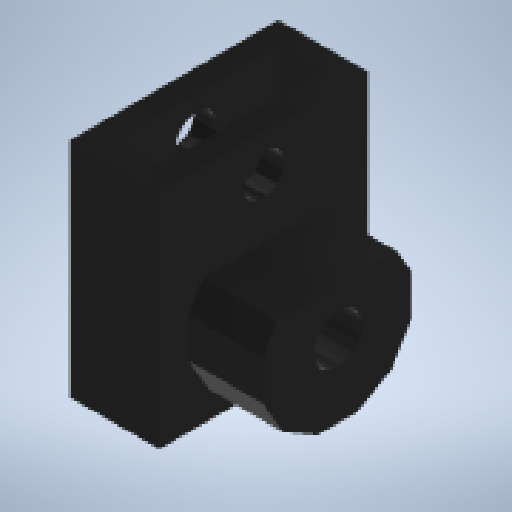
# Autodesk Inventor part: RollY
Saved by Autodesk Inventor 2023 (Build 270158000, 158)
## iProperties
Created: 2023-10-26
Part Number: RollY
Material: Thermoplastic Resin
Document SubType Name: Modeling
Designer: Mustapha
Density: 1.28 g/cm^3
Appearance: Smooth - Black
Mass: 11.287 g
Surface Area: 53.7238 cm^2
Volume: 8.81798 cm^3
Author: Mustapha
Autodesk Inventor part; units mm, degrees
ref_plane "YZ Plane" through (0, 0, 0) normal (1, 0, 0) x (0, 1, 0)
ref_plane "XZ Plane" through (0, 0, 0) normal (0, 1, 0) x (-1, 0, 0)
ref_plane "XY Plane" through (0, 0, 0) normal (0, 0, 1) x (1, 0, 0)
sketch "Sketch1" plane through (0, 0, 0) normal (0, 1, 0) x (-1, 0, 0)
  line L0 (0, 0) -> (6, 0)
  line L1 (6, 0) -> (6, -22)
  line L2 (6, -22) -> (0, -22)
  line L3 (0, -22) -> (0, 0)
  line L4 (9, 3) -> (-3, 3)
  line L5 (-3, 3) -> (-3, -25)
  line L6 (-3, -25) -> (9, -25)
  line L7 (9, -25) -> (9, 3)
  point P0 (3, 0)
  point P1 (3, -25)
  dimension "d0" = 22
  dimension "d1" = 6
  dimension "d2" = 3
  dimension "d3" = 3
  dimension "d4" = 3
  dimension "d5" = 3
  constraints: 16 end point, 4 parallel, 2 horizontal, 2 midpoint, 2 perpendicular
  measures "d0" distance between parallel lines of L2 L0
  measures "d1" distance between parallel lines of L3 L1
  measures "d2" distance from line of L4 point (3, 0)
  measures "d3" distance from line of point (3, -25) L2
  measures "d4" distance between parallel lines of L1 L7
  measures "d5" distance between parallel lines of L5 L3
extrude "Extrusion1" add sketch "Sketch1" along normal blind 30
sketch "Sketch2" plane through (3, 0, 3) normal (1, 0, 0) x (0, 0, -1)
  circle A0 centre (14, 25) radius 2.75
  line L0 (0, 30) -> (28, 30) projected
  point P0 (3, 0)
  dimension "d8" = 5.5
  dimension "d11" = 5
  constraints: 1 centre point
  measures "d8" diameter of A0
  measures "d11" distance from line of A0.centre L0
extrude "Extrusion2" cut sketch "Sketch2" against normal blind 30
sketch "Sketch3" plane through (3, 0, 3) normal (1, 0, 0) x (0, 0, -1)
  line L0 (6.6175, 3.6795) -> (3.938, 8.3205)
  line L1 (3.938, 8.3205) -> (3.938, 13.6795)
  line L2 (3.938, 13.6795) -> (6.6175, 18.3205)
  line L3 (6.6175, 18.3205) -> (11.2585, 21)
  line L4 (11.2585, 21) -> (16.6175, 21)
  line L5 (16.6175, 21) -> (21.2585, 18.3205)
  line L6 (21.2585, 18.3205) -> (23.938, 13.6795)
  line L7 (23.938, 13.6795) -> (23.938, 8.3205)
  line L8 (23.938, 8.3205) -> (21.2585, 3.6795)
  line L9 (21.2585, 3.6795) -> (16.6175, 1)
  line L10 (16.6175, 1) -> (11.2585, 1)
  line L11 (11.2585, 1) -> (6.6175, 3.6795)
  line L12 (0, 30) -> (28, 30) projected
  circle A0 centre (14, 10.8347) radius 3.253
  point P0 (3, 0)
  point P1 (13.938, 11)
  dimension "d12" = 10
  dimension "d13" = 19
  constraints: 24 end point, 1 centre point, 1 parallel, 25 other
  measures "d12" vertical distance of point (13.938, 11) L4.end
  measures "d13" distance from line of L12 point (13.938, 11)
extrude "Extrusion3" add sketch "Sketch3" along normal blind 10
sketch "Sketch5" plane through (3, 10.8347, -11) normal (1, 0, 0) x (0, 0, -1)
  circle A0 centre (0, 0) radius 1.5
  point P0 (-11, -10.8347)
  dimension "d18" = 3
  constraints: 1 centre point
  measures "d18" diameter of A0
extrude "Extrusion5" cut sketch "Sketch5" against normal blind 12
sketch "Sketch6" plane through (13, 0, 3) normal (1, 0, 0) x (0, 0, -1)
  line L0 (23, 22) -> (5, 22)
  line L1 (5, 22) -> (5, 17)
  line L2 (5, 17) -> (23, 17)
  line L3 (23, 17) -> (23, 22)
  line L4 (28, 0) -> (28, 30) projected
  line L5 (0, 0) -> (0, 30) projected
  line L6 (0, 30) -> (28, 30) projected
  point P0 (3, 0)
  dimension "d21" = 5
  dimension "d22" = 5
  dimension "d23" = 5
  dimension "d24" = 8
  constraints: 8 end point, 2 parallel, 1 horizontal, 1 perpendicular
  measures "d21" distance between parallel lines of L3 L4
  measures "d22" distance between parallel lines of L5 L1
  measures "d23" distance between parallel lines of L0 L2
  measures "d24" distance between parallel lines of L6 L0
extrude "Extrusion6" cut sketch "Sketch6" against normal blind 10
equation "\"d22\" = d21"
body "Solid1"
